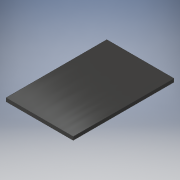
# Autodesk Inventor part: Electr_
Saved by Autodesk Inventor 2019 (Build 230136000, 136)
## iProperties
Created: 2018-11-16
Part Number: Electr_
Material: Generic
Document SubType Name: Modeling
Designer: xwermter
Density: 1 g/cm^3
Appearance: Default
Author: xwermter
Autodesk Inventor part; units mm, degrees
ref_plane "YZ Plane" through (0, 0, 0) normal (1, 0, 0) x (0, 1, 0)
ref_plane "XZ Plane" through (0, 0, 0) normal (0, 1, 0) x (-1, 0, 0)
ref_plane "XY Plane" through (0, 0, 0) normal (0, 0, 1) x (1, 0, 0)
sketch "Sketch1" plane through (0, 0, 0) normal (0, 1, 0) x (-1, 0, 0)
  line L0 (50, 75) -> (-50, 75)
  line L1 (-50, 75) -> (-50, -75)
  line L2 (-50, -75) -> (50, -75)
  line L3 (50, -75) -> (50, 75)
  point P0 (0, 0)
  dimension "d0" = 100
  dimension "d1" = 150
  dimension "d2" = 75
  dimension "d3" = 50
  constraints: 8 end point, 2 parallel, 1 horizontal, 1 perpendicular
  measures "d0" distance of L1.end L2.end
  measures "d1" distance of L2.end L0.start
  measures "d2" distance from line of L2 point (0, 0)
  measures "d3" distance from line of L1 point (0, 0)
extrude "Extrusion1" add sketch "Sketch1" along normal blind 5
body "Solid1"
